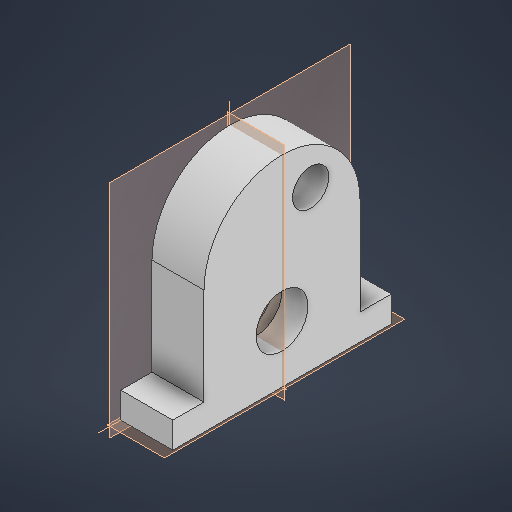
# Autodesk Inventor part: Part1
Saved by Autodesk Inventor 2027.1 (Build 311270010, 270A)
## iProperties
Created: 2026-09-09
Part Number: Part1
Material: Generic
Document SubType Name: Modeling
Designer: thiag
Density: 1 g/cm^3
Appearance: Default
Author: thiag
Autodesk Inventor part; units mm, degrees
sketch "Sketch1" plane through (0, 0, 0) normal (1, 0, 0) x (0, 1, 0)
  circle A0 centre (30.5, -5.5) radius 3.5
  line L0 (11, 15) -> (5, 15)
  line L1 (5, -15) -> (11, -15)
  line L2 (0, -21) -> (5, -21)
  line L3 (5, -21) -> (5, -15)
  line L4 (0, 21) -> (5, 21)
  line L5 (5, 21) -> (5, 15)
  line L6 (-7.7302, 0) -> (46.3815, 0) projected
  line L7 (0, 29.4) -> (0, -29.4) projected
  line L8 (0, 21) -> (0, -21)
  line L9 (11, -15) -> (23.6512, -15)
  line L10 (11, 15) -> (23.6512, 15)
  arc A1 (23.6512, -15) -> (23.6512, 15) centre (23.6512, 0) ccw
  circle A2 centre (11, 0) radius 5
  point P0 (2.5, -21)
  dimension "d7" = 7
  dimension "d45" = 21
  dimension "d64" = 5
  dimension "d65" = 21
  dimension "d66" = 5
  dimension "d67" = 15
  dimension "d69" = 5.5
  dimension "d73" = 0
  dimension "d74" = 30.5
  dimension "d75" = 10
  dimension "d76" = 0
  dimension "d77" = 11
  dimension "d78" = 15
  dimension "d79" = 15
  dimension "d80" = 23.6512
  constraints: 18 end point, 3 centre point, 3 horizontal, 2 point on circle, 1 midpoint, 1 parallel, 1 point on line
  measures "d7" diameter of A0
  measures "d45" distance between parallel lines of L6 L2
  measures "d64" distance between parallel lines of L7 L3
  measures "d65" distance between parallel lines of L4 L6
  measures "d66" distance between parallel lines of L7 L5
  measures "d67" distance from line of L6 L1.start
  measures "d69" distance from line of A0.centre L6
  measures "d73" distance between parallel lines of L7 L8
  measures "d74" distance from line of L8 A0.centre
  measures "d75" diameter of A2
  measures "d76" distance from line of L6 A2.centre
  measures "d77" distance from line of L8 A2.centre
  measures "d78" distance between parallel lines of L6 L10
  measures "d79" radius of A1
  measures "d80" distance from line of L8 A1.centre
extrude "Extrusion1" add sketch "Sketch1" along normal blind 10 contours L10 A1 L6 A2 L7 L4 L5 L0 | A1 L9 L1 L3 L2 L7 L6 A2
sketch "Sketch4" plane through (10, 0, 0) normal (1, 0, 0) x (0, 0, -1)
  circle A0 centre (0, 11) radius 9.5
  circle A1 centre (5.5, 30.5) radius 5
  line L0 (-29.4, 0) -> (29.4, 0) projected
  line L1 (0, -7.7302) -> (0, 46.3815) projected
  point P0 (0, 0)
  dimension "d56" = 19
  dimension "d57" = 10
  dimension "d58" = 11
  dimension "d59" = 0
  dimension "d60" = 30.5
  dimension "d61" = 5.5
  constraints: 2 centre point
  measures "d56" diameter of A0
  measures "d57" diameter of A1
  measures "d58" distance from line of L0 A0.centre
  measures "d59" distance from line of L1 A0.centre
  measures "d60" distance from line of L0 A1.centre
  measures "d61" distance from line of L1 A1.centre
extrude "Extrusion2" cut sketch "Sketch4" along normal blind 5 from surface at -10
body "Solid1"
